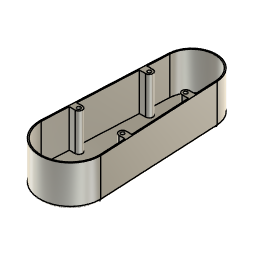
TRARM02_Link3B_100x50x33 (Autodesk Fusion 360 design; units mm, degrees)
Autodesk Fusion 360 part; units mm, degrees
sketch "스케치1" plane through (0, 0, 0) normal (0, 0, 1) x (1, 0, 0)
  line L0 (19.975293, 100.993823) -> (25, 0)
  line L1 (-19.975293, 100.993823) -> (-25, 0)
  arc A0 (19.975293, 100.993823) -> (-19.975293, 100.993823) centre (0, 100) ccw
  arc A1 (-25, 0) -> (25, 0) centre (0, 0) ccw
  dimension "d1" = 50
  dimension "d222" = 20
  dimension "d223" = 100
  constraint coincident A1.centre origin
  constraint tangent L1 A0
  constraint horizontal A1.centre L1.end
  constraint horizontal A1.centre L0.end
  constraint vertical A1.centre A0.centre
  constraint tangent L0 A0
  measures "d1" diameter of A1
  measures "d222" radius of A0
  measures "d223" distance of A1.centre A0.centre
extrude "돌출1" add sketch "스케치1" along normal blind 2
sketch "스케치2" plane through (0, 0, 2) normal (0, 0, 1) x (-1, 0, 0)
  line L0 (19.975293, -100.993823) -> (25, 0)
  arc A0 (-19.975293, -100.993823) -> (19.975293, -100.993823) centre (0, -100) ccw
  line L1 (-25, 0) -> (-19.975293, -100.993823)
  arc A1 (25, 0) -> (-25, 0) centre (0, 0) ccw
  arc A2 (23.998763, 0) -> (-23.998763, 0) centre (0, 0) ccw
  arc A3 (-18.976528, -100.944132) -> (18.976528, -100.944132) centre (0, -100) ccw
  line L2 (-15, -76.999999) -> (-20.167811, -76.999999)
  line L3 (-15, -83.000001) -> (-19.869296, -83.000001)
  line L4 (15, -77.000001) -> (20.167811, -77.000001)
  line L5 (15, -82.999999) -> (19.869296, -82.999999)
  arc A4 (15, -77.000001) -> (15, -82.999999) centre (15, -80) ccw
  line L6 (18.976528, -100.944132) -> (19.869296, -82.999999)
  line L7 (-19.869296, -83.000001) -> (-18.976528, -100.944132)
  arc A5 (-15, -83.000001) -> (-15, -76.999999) centre (-15, -80) ccw
  line L8 (-18, -28) -> (-22.60569, -28)
  line L9 (-18, -22) -> (-22.904205, -22)
  line L10 (18, -28) -> (22.60569, -28)
  line L11 (18, -22) -> (22.904205, -22)
  arc A6 (18, -22) -> (18, -28) centre (18, -25) ccw
  line L12 (20.167811, -77.000001) -> (22.60569, -28)
  line L13 (22.904205, -22) -> (23.998763, 0)
  line L14 (-23.998763, 0) -> (-22.904205, -22)
  line L15 (-22.60569, -28) -> (-20.167811, -76.999999)
  arc A7 (-18, -28) -> (-18, -22) centre (-18, -25) ccw
  dimension "d241" = 6
  dimension "d242" = 15
  dimension "d243" = 15
  dimension "d245" = 25
  dimension "d246" = 18
  dimension "d247" = 18
  dimension "d255" = 20
  constraint equal A6 A7
  constraint equal A5 A7
  constraint equal A4 A5
  constraint horizontal A7.centre A6.centre
  constraint horizontal A5.centre A4.centre
  constraint horizontal L2
  constraint parallel L2 L3
  constraint parallel L3 L4
  constraint parallel L4 L5
  constraint concentric A1 A2
  constraint concentric A0 A3
  constraint tangent A3 L14
  constraint tangent A3 L6
  constraint collinear L6 L12
  constraint collinear L7 L14
  constraint horizontal L8
  constraint coincident L9.start A7
  constraint parallel L8 L9
  constraint parallel L9 L10
  constraint parallel L10 L11
  constraint collinear L12 L13
  constraint collinear L14 L15
  constraint coincident L9 A7.end
  constraint vertical A7.centre L8.start
  constraint vertical A7.centre L9.start
  constraint vertical A6.centre L10.start
  constraint vertical A6.centre L11.start
  measures "d241" diameter of A7
  measures "d242" horizontal distance of A1.centre A5.centre
  measures "d243" horizontal distance of A1.centre A4.centre
  measures "d245" vertical distance of A1.centre A7.centre
  measures "d246" horizontal distance of A1.centre A7.centre
  measures "d247" horizontal distance of A1.centre A6.centre
  measures "d255" vertical distance of A0.centre A5.centre
extrude "돌출29" add sketch "스케치2" along normal blind 31
sketch "스케치26" plane through (0, 0, 33) normal (0, 0, 1) x (-1, 0, 0)
  circle A0 centre (18, -25) radius 1.45
  arc A1 (18, -22) -> (18, -28) centre (18, -25) ccw
  circle A2 centre (-18, -25) radius 1.45
  arc A3 (-18, -28) -> (-18, -22) centre (-18, -25) ccw
  circle A4 centre (15, -80) radius 1.45
  arc A5 (15, -77.000001) -> (15, -82.999999) centre (15, -80) ccw
  circle A6 centre (-15, -80) radius 1.45
  arc A7 (-15, -83.000001) -> (-15, -76.999999) centre (-15, -80) ccw
  dimension "d248" = 2.9
  constraint concentric A0 A1
  constraint concentric A2 A3
  constraint concentric A4 A5
  constraint concentric A6 A7
  constraint equal A4 A6
  constraint equal A0 A6
  constraint equal A0 A2
  measures "d248" diameter of A0
extrude "돌출30" cut sketch "스케치26" against normal blind 5
fillet "필렛6" radius 2 4 edges at (0, -25, 0) (-22.487646, 50.496912, 0) (0, 120, 0) (22.487646, 50.496912, 0)
